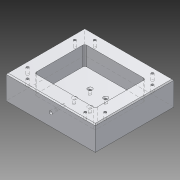
# Autodesk Inventor part: UNLHEP-14-01-P-002_ChuckForBonder
Saved by Autodesk Inventor 2013 (Build 170138000, 138)
## iProperties
Created: 2014-01-09
Part Number: UNLHEP-14-01-P-002_ChuckForBonder
Material: Aluminium 6061
Document SubType Name: Modeling
Designer: Frank Meier
Density: 2.71 g/cm^3
Project: UNL Pixel Phase I
Description: ChuckForBonder
Mass: 2082.68 g
Surface Area: 968.267 cm^2
Volume: 768.515 cm^3
Author: Frank Meier
Revision Number: 00
Autodesk Inventor part; units mm, degrees
ref_plane "YZ Plane" through (0, 0, 0) normal (1, 0, 0) x (0, 1, 0)
ref_plane "XZ Plane" through (0, 0, 0) normal (0, 1, 0) x (-1, 0, 0)
ref_plane "XY Plane" through (0, 0, 0) normal (0, 0, 1) x (1, 0, 0)
sketch "Skizze1" plane through (0, 0, 0) normal (0, 0, 1) x (1, 0, 0)
  line L0 (-85, -75) -> (85, -75)
  line L1 (85, -75) -> (85, 75)
  line L2 (85, 75) -> (-85, 75)
  line L3 (-85, 75) -> (-85, -75)
  line L4 (-85, -75) -> (85, 75) construction
  line L5 (85, -75) -> (-85, 75) construction
  point P0 (0, 0)
  dimension "d0" = 170
  dimension "d2" = 150
  constraints: 12 end point, 2 midpoint, 2 parallel, 1 horizontal, 1 perpendicular
  measures "d0" distance of L1.end L2.end
  measures "d2" distance of L0.end L1.end
extrude "Extrusion1" add sketch "Skizze1" along normal blind 46
sketch "Skizze2" plane through (0, 0, 46) normal (0, 0, 1) x (1, 0, 0)
  line L0 (-58, -48) -> (58, -48)
  line L1 (58, -48) -> (58, 48)
  line L2 (58, 48) -> (-58, 48)
  line L3 (-58, 48) -> (-58, -48)
  line L4 (-58, -48) -> (58, 48) construction
  line L5 (58, -48) -> (-58, 48) construction
  line L6 (-85, -75) -> (85, -75) projected
  line L7 (85, -75) -> (85, 75) projected
  line L8 (85, 75) -> (-85, 75) projected
  line L9 (-85, 75) -> (-85, -75) projected
  circle A0 centre (-77, 45) radius 2
  circle A1 centre (-55, 67) radius 2
  circle A2 centre (55, 67) radius 2
  circle A3 centre (77, 45) radius 2
  circle A4 centre (77, -45) radius 2
  circle A5 centre (55, -67) radius 2
  circle A6 centre (-55, -67) radius 2
  circle A7 centre (-77, -45) radius 2
  point P0 (0, 0)
  dimension "d5" = 116
  dimension "d7" = 96
  dimension "d14" = 8
  dimension "d15" = 30
  dimension "d16" = 30
  dimension "d17" = 8
  dimension "d18" = 8
  dimension "d19" = 30
  dimension "d20" = 8
  dimension "d21" = 30
  dimension "d22" = 30
  dimension "d23" = 8
  dimension "d24" = 8
  dimension "d25" = 30
  dimension "d26" = 8
  dimension "d27" = 30
  dimension "d28" = 30
  dimension "d29" = 8
  dimension "d30" = 4
  dimension "d31" = 4
  dimension "d32" = 4
  dimension "d33" = 4
  dimension "d34" = 4
  dimension "d35" = 4
  dimension "d36" = 4
  dimension "d37" = 4
  constraints: 12 end point, 8 centre point, 8 coincident, 2 midpoint, 2 parallel, 1 horizontal, 1 perpendicular
  measures "d5" distance of L1.end L2.end
  measures "d7" distance of L0.end L1.end
  measures "d14" distance from line of L9 point (-77, 45)
  measures "d15" distance from line of L8 point (-77, 45)
  measures "d16" distance from line of L9 point (-55, 67)
  measures "d17" distance from line of L8 point (-55, 67)
  measures "d18" distance from line of L8 point (55, 67)
  measures "d19" distance from line of L7 point (55, 67)
  measures "d20" distance from line of L7 point (77, 45)
  measures "d21" distance from line of L8 point (77, 45)
  measures "d22" distance from line of L6 point (77, -45)
  measures "d23" distance from line of L7 point (77, -45)
  measures "d24" distance from line of L6 point (55, -67)
  measures "d25" distance from line of L7 point (55, -67)
  measures "d26" distance from line of L6 point (-55, -67)
  measures "d27" distance from line of L9 point (-55, -67)
  measures "d28" distance from line of L6 point (-77, -45)
  measures "d29" distance from line of L9 point (-77, -45)
  measures "d30" diameter of A0
  measures "d31" diameter of A1
  measures "d32" diameter of A2
  measures "d33" diameter of A3
  measures "d34" diameter of A4
  measures "d35" diameter of A5
  measures "d36" diameter of A6
  measures "d37" diameter of A7
extrude "Extrusion2" cut sketch "Skizze2" against normal blind 36 contours L3 L2 L1 L0
fillet "Rundung1" radius 4 4 edges at (-58, 48, 28) (58, 48, 28) (58, -48, 28) (-58, -48, 28)
chamfer "Fase1" distance 2 angle 45 4 edges at (0, -75, 46) (-85, 0, 46) (0, 75, 46) (85, 0, 46)
sketch "Skizze4" plane through (0, 0, 46) normal (0, 0, 1) x (1, 0, 0)
  circle A0 centre (-74, 45) radius 2.25
  circle A1 centre (-55, 64) radius 2.25
  circle A2 centre (55, 64) radius 2.25
  circle A3 centre (74, 45) radius 2.25
  circle A4 centre (74, -45) radius 2.25
  circle A5 centre (55, -64) radius 2.25
  circle A6 centre (-55, -64) radius 2.25
  circle A7 centre (-74, -45) radius 2.25
  line L0 (85, -75) -> (85, 75) projected
  line L1 (-85, 75) -> (-85, -75) projected
  line L2 (85, 75) -> (-85, 75) projected
  line L3 (-85, -75) -> (85, -75) projected
  dimension "d56" = 4.5
  dimension "d57" = 4.5
  dimension "d58" = 4.5
  dimension "d59" = 4.5
  dimension "d60" = 4.5
  dimension "d61" = 4.5
  dimension "d62" = 4.5
  dimension "d63" = 4.5
  dimension "d92" = 30
  dimension "d93" = 30
  dimension "d94" = 11
  dimension "d95" = 11
  dimension "d96" = 11
  dimension "d97" = 11
  dimension "d98" = 148
  dimension "d99" = 30
  dimension "d100" = 30
  dimension "d101" = 11
  dimension "d102" = 11
  dimension "d103" = 11
  dimension "d104" = 11
  dimension "d105" = 128
  dimension "d106" = 128
  dimension "d107" = 30
  dimension "d108" = 30
  dimension "d109" = 30
  dimension "d110" = 30
  constraints: 8 centre point, 8 coincident
  measures "d56" diameter of A0
  measures "d57" diameter of A1
  measures "d58" diameter of A2
  measures "d59" diameter of A3
  measures "d60" diameter of A4
  measures "d61" diameter of A5
  measures "d62" diameter of A6
  measures "d63" diameter of A7
  measures "d92" distance from line of L0 A2.centre
  measures "d93" distance from line of L1 A1.centre
  measures "d94" distance from line of L0 A3.centre
  measures "d95" distance from line of L1 A0.centre
  measures "d96" distance from line of L1 A7.centre
  measures "d97" distance from line of L0 A4.centre
  measures "d98" distance of point (74, 45) A0.centre
  measures "d99" distance from line of L2 A0.centre
  measures "d100" distance from line of L2 A3.centre
  measures "d101" distance from line of L2 point (55, 64)
  measures "d102" distance from line of L2 A1.centre
  measures "d103" distance from line of L3 A6.centre
  measures "d104" distance from line of L3 A5.centre
  measures "d105" distance of point (-55, 64) point (-55, -64)
  measures "d106" distance of point (55, -64) point (55, 64)
  measures "d107" distance from line of L0 point (55, -64)
  measures "d108" distance from line of L1 point (-55, -64)
  measures "d109" distance from line of L3 point (-74, -45)
  measures "d110" distance from line of L3 point (74, -45)
extrude "Extrusion4" cut sketch "Skizze4" against normal blind 12 contours A0 | A1 | A2 | A3 | A4 | A5 | A6 | A7
sketch "Skizze5" plane through (0, 0, 10) normal (0, 0, 1) x (1, 0, 0)
  point P0 (0, 0)
  point P1 (15, 15)
  point P2 (15, -15)
  point P3 (-15, -15)
  point P4 (-15, 15)
  dimension "d68" = 15
  dimension "d69" = 15
  dimension "d70" = 30
  dimension "d71" = 30
  dimension "d72" = 30
  dimension "d73" = 30
  dimension "d74" = 15
  dimension "d75" = 15
  measures "d68" horizontal distance of point (0, 0) point (15, 15)
  measures "d69" horizontal distance of point (0, 0) point (15, 15)
  measures "d70" distance of point (15, 15) point (-15, 15)
  measures "d71" distance of point (15, 15) point (15, -15)
  measures "d72" distance of point (-15, -15) point (-15, 15)
  measures "d73" distance of point (15, -15) point (-15, -15)
  measures "d74" horizontal distance of point (0, 0) point (-15, 15)
  measures "d75" horizontal distance of point (0, 0) point (15, -15)
hole "Bohrung1" at (15, 15, 10) at (15, -15, 10) at (-15, -15, 10) at (-15, 15, 10) direction (0, 0, -1) diameter 4.5 depth 15 tip angle 118 countersink diameter 8.6 countersink angle 90
sketch "Skizze7" plane through (-85, -75, 0) normal (0, -1, 0) x (1, 0, 0)
  line L0 (0, 0) -> (0, 44) projected
  point P0 (85, 0)
  point P1 (85, 23)
  dimension "d83" = 23
  dimension "d84" = 85
  measures "d83" distance of point (85, 0) point (85, 23)
  measures "d84" distance from line of L0 point (85, 23)
hole "Bohrung2" at (0, -75, 23) direction (0, 1, 0) diameter 4 depth 30 tip angle 118 counterbore diameter 6 counterbore depth 10
